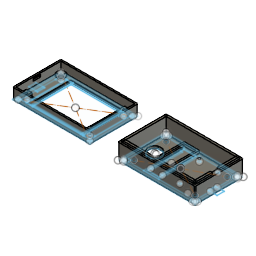
dcdc_cases (Autodesk Fusion 360 design; units mm, degrees)
part number: 2026-03-09-11-10-45-876
Autodesk Fusion 360 part; units mm, degrees
sketch "Sketch1" plane through (0, 0, 0) normal (0, 1, 0) x (1, 0, 0)
  line L0 (0, 0) -> (30.8, 0)
  line L1 (30.8, 0) -> (30.8, 45.2)
  line L2 (30.8, 45.2) -> (0, 45.2)
  line L3 (0, 45.2) -> (0, 0)
  line L4 (0, 0) -> (30.8, 0)
  line L5 (30.8, 0) -> (30.8, 37.2)
  line L6 (30.8, 37.2) -> (0, 37.2)
  line L7 (0, 37.2) -> (0, 0)
  line L8 (0, 45.2) -> (3.78, 45.2)
  line L9 (0, 41.42) -> (0, 45.2)
  circle A0 centre (3.78, 41.42) radius 1.85
  circle A1 centre (27, 41.42) radius 1.85
  line L10 (15.4, 0) -> (0, 0)
  line L11 (0, 0) -> (0, 5.5)
  circle A2 centre (15.4, 5.5) radius 2
  circle A3 centre (15.4, 5.5) radius 3
  line L12 (-1.5, 0) -> (-1.5, 45.2)
  line L13 (-1.5, 45.2) -> (0, 45.2)
  line L14 (0, 45.2) -> (0, 0)
  line L15 (32.3, 0) -> (32.3, 45.2)
  line L16 (32.3, 45.2) -> (30.8, 45.2)
  line L17 (30.8, 45.2) -> (30.8, 0)
  line L18 (32.3, 0) -> (32.3, -1.5)
  line L19 (32.3, -1.5) -> (-1.5, -1.5)
  line L20 (-1.5, -1.5) -> (-1.5, 0)
  circle A4 centre (40.4187, 7.745) radius 3
  circle A5 centre (40.4187, 7.745) radius 2
  line L21 (30.8, 44.0804) -> (30.8, 41.0217)
  line L22 (-1.5, 45.2) -> (32.3, 45.2)
  line L23 (32.3, 45.2) -> (32.3, -1.5)
  line L24 (32.3, -1.5) -> (-1.5, -1.5)
  line L25 (-1.5, -1.5) -> (-1.5, 45.2)
  circle A6 centre (40.4187, 7.745) radius 3
  line L26 (15.4, 0) -> (0, 0)
  line L27 (30.8, 0) -> (30.8, 45.2)
  line L28 (30.8, 44.0804) -> (30.8, 41.0217)
  line L29 (32.3, 0) -> (32.3, 45.2)
  line L30 (30.8, 0) -> (30.8, 37.2)
  line L31 (32.3, 45.2) -> (30.8, 45.2)
  line L32 (30.8, 45.2) -> (0, 45.2)
  line L33 (32.3, 0) -> (32.3, -1.5)
  line L34 (0, 0) -> (30.8, 0)
  line L35 (30.8, 45.2) -> (30.8, 0)
  circle A7 centre (15.4, 5.5) radius 2
  line L36 (30.8, 37.2) -> (0, 37.2)
  line L37 (32.3, 45.2) -> (32.3, -1.5)
  line L38 (0, 0) -> (0, 5.5)
  line L39 (-1.5, 45.2) -> (32.3, 45.2)
  line L40 (0, 37.2) -> (0, 0)
  line L41 (32.3, -1.5) -> (-1.5, -1.5)
  line L42 (0, 0) -> (30.8, 0)
  line L43 (32.3, -1.5) -> (-1.5, -1.5)
  line L44 (-1.5, -1.5) -> (-1.5, 45.2)
  line L45 (-1.5, 0) -> (-1.5, 45.2)
  line L46 (0, 45.2) -> (0, 0)
  circle A8 centre (40.4187, 7.745) radius 2
  line L47 (0, 45.2) -> (0, 0)
  circle A9 centre (27, 41.42) radius 1.85
  circle A10 centre (15.4, 5.5) radius 3
  line L48 (-1.5, -1.5) -> (-1.5, 0)
  circle A11 centre (3.78, 41.42) radius 1.85
  line L49 (0, 41.42) -> (0, 45.2)
  line L50 (0, 45.2) -> (3.78, 45.2)
  line L51 (-1.5, 45.2) -> (0, 45.2)
  dimension "d7" = 3.7
  dimension "d8" = 3.7
  dimension "d10" = 4
  dimension "d11" = 6
  dimension "d12" = 1.5
  dimension "d13" = 1.5
  dimension "d14" = 1.5
  dimension "d50" = 6
  dimension "d51" = 4
  dimension "d79" = 33.8
  dimension "d80" = 46.7
  dimension "d127" = 3.7
  dimension "d128" = 3.7
  dimension "d129" = 4
  dimension "d130" = 6
  dimension "d131" = 1.5
  dimension "d132" = 1.5
  dimension "d133" = 1.5
  dimension "d134" = 6
  dimension "d135" = 4
  dimension "d136" = 33.8
  dimension "d137" = 46.7
  constraint horizontal L0
  constraint vertical L1
  constraint horizontal L2
  constraint vertical L3
  constraint coincident L0.start L3.end
  constraint horizontal L4
  constraint vertical L5
  constraint horizontal L6
  constraint vertical L7
  constraint horizontal L8
  constraint vertical L9
  constraint horizontal L10
  constraint vertical L11
  constraint midpoint L4 L10.start
  constraint concentric A2 A3
  constraint vertical L12
  constraint horizontal L13
  constraint vertical L14
  constraint vertical L15
  constraint horizontal L16
  constraint vertical L17
  constraint vertical L18
  constraint horizontal L19
  constraint vertical L20
  constraint concentric A4 A5
  constraint vertical L21
  constraint coincident L17 L21.end
  constraint horizontal L22
  constraint vertical L23
  constraint horizontal L24
  constraint vertical L25
  constraint horizontal L34
  constraint vertical L27
  constraint horizontal L32
  constraint vertical L46
  constraint horizontal L42
  constraint vertical L30
  constraint horizontal L36
  constraint vertical L40
  constraint horizontal L50
  constraint vertical L49
  constraint horizontal L26
  constraint vertical L38
  constraint midpoint L10.start L42
  constraint concentric A7 A10
  constraint vertical L45
  constraint horizontal L51
  constraint vertical L47
  constraint vertical L29
  constraint horizontal L31
  constraint vertical L35
  constraint vertical L33
  constraint horizontal L43
  constraint vertical L48
  constraint concentric A6 A8
  constraint vertical L28
  constraint coincident L21.end L35
  constraint horizontal L39
  constraint vertical L37
  constraint horizontal L41
  constraint vertical L44
  measures "d7" diameter of A0
  measures "d8" diameter of A1
  measures "d10" diameter of A2
  measures "d11" diameter of A3
  measures "d12" distance of L0.start L12.start
  measures "d13" distance of L0.end L15.start
  measures "d14" distance of L12.start L19.end
  measures "d50" diameter of A4
  measures "d51" diameter of A5
  measures "d79" distance of L18.end L19.end
  measures "d80" distance of L12.end L19.end
  measures "d127" diameter of A11
  measures "d128" diameter of A9
  measures "d129" diameter of A7
  measures "d130" diameter of A10
  measures "d131" distance of L0.start L12.start
  measures "d132" distance of L0.end L15.start
  measures "d133" distance of L19.end L12.start
  measures "d134" diameter of A6
  measures "d135" diameter of A8
  measures "d136" distance of L19.end L18.end
  measures "d137" distance of L19.end L12.end
extrude "Extrude1" add sketch "Sketch1" along normal blind 1.5 contours L0 L1 L3 L4 L5 L6 L7 L10 L11 L14 L17 L26 L27 L30 L34 L35 L36 L38 L40 L42 L46 L47 | L1 L2 L3 L6 L8 L9 L14 L17 L21 L22 L27 L28 L32 L35 L36 L39 L46 L47 L49 L50 | A3 A10 makes body 1
extrude "Extrude2" add sketch "Sketch1" along normal blind 17.7 contours L0 L1 L3 L4 L5 L7 L9 L10 L11 L12 L13 L14 L15 L16 L17 L18 L19 L20 L21 L22 L23 L24 L25 L26 L27 L28 L29 L30 L31 L33 L34 L35 L37 L38 L39 L40 L41 L42 L43 L44 L45 L46 L47 L48 L49 L51 bodies 1
ref_plane "WorkPlane1" through (15.4, 17.7, -21.85) normal (0, 1, 0) x (0, 0, 1)
sketch "Sketch2" plane through (0, 17.7, 0) normal (0, 1, 0) x (1, 0, 0)
  line L0 (-1.5, -1.5) -> (32.3, -1.5)
  line L1 (32.3, -1.5) -> (32.3, 37.2)
  line L2 (32.3, 37.2) -> (-1.5, 37.2)
  line L3 (-1.5, 37.2) -> (-1.5, -1.5)
  circle A0 centre (15.4, 5.5) radius 2
  circle A1 centre (15.4, 5.5) radius 3
  dimension "d20" = 4
  dimension "d21" = 6
  constraint horizontal L0
  constraint vertical L1
  constraint horizontal L2
  constraint vertical L3
  constraint concentric A0 A1
  measures "d20" diameter of A0
  measures "d21" diameter of A1
extrude "Extrude3" add sketch "Sketch2" along normal blind 1.5 contours L0 L1 L2 L3 bodies 1
fillet "Fillet1" radius 1 2 edges at (31.55, 17.7, -37.2) (-0.75, 17.7, -37.2) on bodies 1
fillet "Fillet2" radius 2 2 edges at (-0.75, 17.7, -45.2) (31.55, 17.7, -45.2) on bodies 1
sketch "mini-170" plane through (0, 0, 0) normal (0, 1, 0) x (1, 0, 0)
  line L0 (0, 0) -> (10.9, 0)
  line L1 (10.9, 0) -> (10.9, 20.2)
  line L2 (0, 20.2) -> (0, 0)
  line L3 (-1.5, 20.2) -> (-1.5, 0)
  line L4 (0, 0) -> (0, 20.2)
  line L5 (12.4, 20.2) -> (12.4, 0)
  line L6 (10.9, 0) -> (10.9, 20.2)
  line L7 (12.4, 0) -> (12.4, -1.5)
  line L8 (12.4, -1.5) -> (-1.5, -1.5)
  line L9 (-1.5, -1.5) -> (-1.5, 0)
  line L10 (-1.5, 9.9832) -> (-1.5, 11.0323)
  line L11 (-6.4986, 11.0323) -> (-6.4986, 9.9832)
  line L12 (12.4, 10.1) -> (12.4, 11.4359)
  circle A0 centre (-3.9993, 9.9832) radius 1.5
  circle A1 centre (14.9, 10.1) radius 1.5
  arc A2 (-1.5, 15.1) -> (-1.5, 5.1) centre (-1.5, 10.1) ccw
  arc A3 (12.4, 5.1) -> (12.4, 15.1) centre (12.4, 10.1) ccw
  line L13 (12.4, 20.2) -> (12.4, 23.2)
  line L14 (12.4, 23.2) -> (-1.5, 23.2)
  line L15 (-1.5, 23.2) -> (-1.5, 20.2)
  line L16 (-1.5, 20.2) -> (-1.5, 23.2)
  line L17 (-1.5, 23.2) -> (0, 23.2)
  line L18 (0, 23.2) -> (0, 20.2)
  line L19 (12.4, 20.2) -> (12.4, 23.2)
  line L20 (12.4, 23.2) -> (10.9, 23.2)
  line L21 (10.9, 23.2) -> (10.9, 20.2)
  constraint horizontal L0
  constraint vertical L1
  constraint vertical L2
  constraint coincident L0.start L2.end
  constraint vertical L3
  constraint vertical L4
  constraint vertical L5
  constraint vertical L6
  constraint vertical L7
  constraint horizontal L8
  constraint vertical L9
  constraint midpoint L5 L12.start
  constraint midpoint L3 A2.centre
  constraint vertical L10
  constraint vertical L11
  constraint coincident L3 L10.end
  constraint coincident L11.end A2
  constraint vertical L12
  constraint coincident L5 L12.end
  constraint coincident L3 A2.start
  constraint coincident L3 A2.end
  constraint coincident L5 A3.start
  constraint coincident L5 A3.end
  constraint vertical L13
  constraint horizontal L14
  constraint vertical L15
  constraint vertical L16
  constraint horizontal L17
  constraint vertical L18
  constraint vertical L19
  constraint horizontal L20
  constraint vertical L21
extrude "Extrude5" add sketch "mini-170" along normal blind 1.5 separate body contours L0 L1 L2 L4 L6 L14 L18 L21 makes body 2
extrude "Extrude6" add sketch "mini-170" along normal blind 6.1 contours L0 L1 L2 L3 L4 L5 L6 L7 L8 L9 L10 L12 L13 L14 L15 L16 L17 L18 L19 L20 L21 bodies 2
ref_plane "WorkPlane2" through (5.45, 6.1, -10.85) normal (0, 1, 0) x (0, 0, 1)
sketch "mini-170_top" plane through (0, 6.1, 0) normal (0, 1, 0) x (1, 0, 0)
  line L0 (-1.5, -1.5) -> (12.4, -1.5)
  line L1 (12.4, -1.5) -> (12.4, 23.2)
  line L2 (12.4, 23.2) -> (-1.5, 23.2)
  line L3 (-1.5, 23.2) -> (-1.5, -1.5)
  dimension "d45" = 13.9
  constraint horizontal L0
  constraint vertical L1
  constraint horizontal L2
  constraint vertical L3
  measures "d45" distance of L0.start L0.end
extrude "Extrude7" add sketch "mini-170_top" along normal blind 1.5 bodies 2
extrude "Extrude8" add sketch "mini-170" along normal blind 4 contours L3 L10 A2 | L5 L12 A3 bodies 2
extrude "Extrude9" add sketch "Sketch1" along normal blind 15.3 separate body contours A4 A6 makes body 3
sketch "esp_main_board" plane through (0, 0, 0) normal (0, 1, 0) x (1, 0, 0)
  line L0 (91.015, 60.1) -> (-4.985, 60.1)
  line L1 (0, 32.65) -> (0, 23.8)
  line L2 (2, 32.65) -> (0, 32.65)
  circle A0 centre (87.5225, 3.55) radius 1.25
  line L3 (74.83, 55.2) -> (77.53, 55.2)
  circle A1 centre (4, 9) radius 0.9
  line L4 (74.83, 7.7) -> (14.9, 7.7)
  line L5 (0, 55.2) -> (-2.985, 55.2)
  circle A2 centre (87.5225, 56.65) radius 1.25
  line L6 (-2.985, 58.1) -> (0, 58.1)
  line L7 (86.03, 5) -> (77.53, 5)
  line L8 (14.9, 5) -> (74.83, 5)
  line L9 (89.015, 2.1) -> (89.015, 58.1)
  line L10 (77.53, 5) -> (77.53, 55.2)
  line L11 (77.53, 5) -> (74.83, 5)
  line L12 (2, 23.8) -> (2, 32.65)
  line L13 (0, 55.2) -> (0, 5)
  line L14 (77.53, 5) -> (77.53, 55.2)
  line L15 (14.9, 5) -> (14.9, 55.2)
  line L16 (0, 5) -> (-2.985, 5)
  line L17 (86.03, 5) -> (0, 5)
  line L18 (7.03, 5) -> (77.53, 5)
  line L19 (-2.985, 2.1) -> (89.015, 58.1) construction
  circle A3 centre (82.03, 9) radius 0.9
  line L20 (91.015, 0.1) -> (-4.985, 60.1) construction
  line L21 (89.015, 55.2) -> (89.015, 58.1)
  line L22 (-4.985, 0.1) -> (91.015, 0.1)
  line L23 (7.6, 5) -> (14.9, 5)
  line L24 (91.015, 0.1) -> (91.015, 60.1)
  line L25 (14.9, 52.5) -> (14.9, 55.2)
  line L26 (89.015, 2.1) -> (-2.985, 58.1) construction
  line L27 (-2.985, 2.1) -> (89.015, 2.1)
  line L28 (89.015, 2.1) -> (86.03, 2.1)
  line L29 (86.03, 55.2) -> (89.015, 55.2)
  line L30 (86.03, 58.1) -> (86.03, 55.2)
  line L31 (86.03, 2.1) -> (86.03, 5)
  line L32 (77.53, 55.2) -> (77.53, 5)
  line L33 (74.83, 52.5) -> (14.9, 52.5)
  circle A4 centre (82.03, 51.2) radius 0.9
  line L34 (86.03, 55.2) -> (86.03, 5)
  line L35 (74.83, 55.2) -> (74.83, 52.5)
  line L36 (0, 2.1) -> (0, 5)
  line L37 (89.015, 5) -> (89.015, 2.1)
  line L38 (77.53, 55.2) -> (86.03, 55.2)
  line L39 (89.015, 58.1) -> (86.03, 58.1)
  line L40 (86.03, 55.2) -> (86.03, 5)
  line L41 (74.83, 5) -> (74.83, 7.7)
  line L42 (89.015, 58.1) -> (-2.985, 58.1)
  line L43 (0, 58.1) -> (0, 55.2)
  line L44 (7.6, 5) -> (7.6, 55.2)
  line L45 (86.03, 5) -> (89.015, 5)
  line L46 (14.9, 7.7) -> (14.9, 5)
  circle A5 centre (-1.4925, 56.65) radius 1.25
  line L47 (0, 5) -> (7.6, 5)
  line L48 (-2.985, 55.2) -> (-2.985, 58.1)
  line L49 (-2.985, 5) -> (-2.985, 2.1)
  circle A6 centre (4, 51.2) radius 0.9
  line L50 (74.83, 5) -> (74.83, 55.2)
  circle A7 centre (-1.4925, 3.55) radius 1.25
  line L51 (7.03, 55.2) -> (7.03, 5)
  line L52 (-2.985, 2.1) -> (0, 2.1)
  line L53 (14.9, 55.2) -> (74.83, 55.2)
  line L54 (-4.985, 60.1) -> (-4.985, 0.1)
  line L55 (7.6, 55.2) -> (0, 55.2)
  line L56 (-2.985, 58.1) -> (-2.985, 2.1)
  line L57 (7.6, 55.2) -> (7.6, 5)
  line L58 (0, 23.8) -> (2, 23.8)
  line L59 (77.53, 55.2) -> (7.03, 55.2)
  line L60 (-4.985, 0.1) -> (91.015, 60.1) construction
  line L61 (14.9, 55.2) -> (7.6, 55.2)
  line L62 (0, 5) -> (7.03, 5)
  line L63 (7.03, 5) -> (7.03, 12)
  line L64 (7.03, 12) -> (0, 12)
  line L65 (0, 12) -> (0, 5)
  line L66 (0, 55.2) -> (7.03, 55.2)
  line L67 (7.03, 55.2) -> (7.03, 48.2)
  line L68 (7.03, 48.2) -> (0, 48.2)
  line L69 (0, 48.2) -> (0, 55.2)
  line L70 (86.03, 55.2) -> (79.03, 55.2)
  line L71 (79.03, 55.2) -> (79.03, 48.2)
  line L72 (79.03, 48.2) -> (86.03, 48.2)
  line L73 (86.03, 48.2) -> (86.03, 55.2)
  line L74 (86.03, 5) -> (79.03, 5)
  line L75 (79.03, 5) -> (79.03, 12)
  line L76 (79.03, 12) -> (86.03, 12)
  line L77 (86.03, 12) -> (86.03, 5)
  line L78 (2, 23.8) -> (-8.6658, 23.8)
  line L79 (-8.6658, 23.8) -> (-8.6658, 32.65)
  line L80 (-8.6658, 32.65) -> (2, 32.65)
  line L81 (2, 32.65) -> (2, 23.8)
  line L82 (14.9, 55.2) -> (12.2, 55.2)
  line L83 (12.2, 55.2) -> (12.2, 5)
  line L84 (12.2, 5) -> (14.9, 5)
  line L85 (14.9, 5) -> (14.9, 55.2)
  line L86 (14.9, 53.85) -> (76.18, 53.85)
  line L87 (14.9, 53.85) -> (13.55, 53.85)
  line L88 (14.9, 6.35) -> (76.18, 6.35)
  line L89 (14.9, 6.35) -> (13.55, 6.35)
  line L90 (13.55, 6.35) -> (76.18, 6.35)
  line L91 (76.18, 6.35) -> (76.18, 53.85)
  line L92 (13.55, 53.85) -> (13.55, 6.35)
  line L93 (126.015, 0.1) -> (126.015, 60.1)
  line L94 (222.015, 60.1) -> (222.015, 0.1)
  line L95 (138.8674, 22.8706) -> (144.6215, 22.8706)
  line L96 (131, 2.1) -> (131, 5)
  line L97 (131, 58.1) -> (131, 55.2)
  line L98 (131, 5) -> (128.015, 5)
  line L99 (131, 55.2) -> (128.015, 55.2)
  arc A8 (144.6215, 22.8706) -> (144.6215, 37.3706) centre (141.7444, 30.1206) ccw
  line L100 (126.015, 60.1) -> (222.015, 60.1)
  line L101 (222.015, 0.1) -> (126.015, 0.1)
  arc A9 (138.8674, 37.3706) -> (138.8674, 22.8706) centre (141.7444, 30.1206) ccw
  line L102 (144.6215, 37.3706) -> (138.8674, 37.3706)
  circle A10 centre (201.25, 49.42) radius 1.45
  line L103 (225.6958, 23.8) -> (225.6958, 32.65)
  line L104 (215.03, 23.8) -> (225.6958, 23.8)
  line L105 (225.6958, 32.65) -> (215.03, 32.65)
  circle A11 centre (178.03, 49.42) radius 1.45
  circle A12 centre (189.63, 13.5) radius 1.45
  line L106 (217.03, 5) -> (220.015, 5)
  line L107 (215.03, 32.65) -> (217.03, 32.65)
  line L108 (217.03, 2.1) -> (217.03, 5)
  line L109 (217.03, 23.8) -> (215.03, 23.8)
  line L110 (215.03, 23.8) -> (215.03, 32.65)
  line L111 (215.03, 32.65) -> (215.03, 23.8)
  line L112 (217.03, 58.1) -> (217.03, 55.2)
  line L113 (217.03, 55.2) -> (220.015, 55.2)
  line L114 (170, 53) -> (155.3, 53)
  line L115 (155.3, 53) -> (155.3, 7.5)
  line L116 (155.3, 7.5) -> (170, 7.5)
  line L117 (170, 7.5) -> (170, 53)
  line L118 (130.815, 55.3) -> (217.215, 55.3)
  line L119 (217.215, 55.3) -> (217.215, 4.9)
  line L120 (217.215, 4.9) -> (130.815, 4.9)
  line L121 (130.815, 4.9) -> (130.815, 55.3)
  line L122 (128.09, 58.025) -> (219.94, 58.025)
  line L123 (219.94, 58.025) -> (219.94, 2.175)
  line L124 (219.94, 2.175) -> (128.09, 2.175)
  line L125 (128.09, 2.175) -> (128.09, 58.025)
  line L126 (128.09, 58.025) -> (134.09, 58.025)
  line L127 (134.09, 58.025) -> (134.09, 52.025)
  line L128 (134.09, 52.025) -> (128.09, 52.025)
  line L129 (128.09, 52.025) -> (128.09, 58.025)
  line L130 (128.09, 2.175) -> (134.09, 2.175)
  line L131 (134.09, 2.175) -> (134.09, 8.175)
  line L132 (134.09, 8.175) -> (128.09, 8.175)
  line L133 (128.09, 8.175) -> (128.09, 2.175)
  line L134 (219.94, 58.025) -> (213.94, 58.025)
  line L135 (213.94, 58.025) -> (213.94, 52.025)
  line L136 (213.94, 52.025) -> (219.94, 52.025)
  line L137 (219.94, 52.025) -> (219.94, 58.025)
  line L138 (219.94, 2.175) -> (213.94, 2.175)
  line L139 (213.94, 2.175) -> (213.94, 8.175)
  line L140 (213.94, 8.175) -> (219.94, 8.175)
  line L141 (219.94, 8.175) -> (219.94, 2.175)
  line L142 (172.15, 4.9) -> (153.15, 4.9)
  line L143 (153.15, 4.9) -> (153.15, 55.3)
  line L144 (172.15, 55.3) -> (172.15, 4.9)
  line L145 (155.3, 53) -> (170, 53)
  line L146 (170, 53) -> (170, 49)
  line L147 (155.3, 49) -> (155.3, 53)
  line L148 (155.3, 7.5) -> (170, 7.5)
  line L149 (170, 7.5) -> (170, 11.5)
  line L150 (155.3, 11.5) -> (155.3, 7.5)
  line L151 (155.3, 49) -> (157.3, 49)
  line L152 (157.3, 49) -> (157.3, 11.5)
  line L153 (157.3, 11.5) -> (155.3, 11.5)
  line L154 (155.3, 11.5) -> (155.3, 49)
  line L155 (170, 49) -> (168, 49)
  line L156 (168, 49) -> (168, 11.5)
  line L157 (168, 11.5) -> (170, 11.5)
  line L158 (170, 11.5) -> (170, 49)
  circle A13 centre (129.5075, 56.65) radius 1.4
  circle A14 centre (218.5225, 56.65) radius 1.4
  circle A15 centre (129.5075, 3.55) radius 1.4
  circle A16 centre (218.5225, 3.55) radius 1.45
  line L159 (212.015, 10.1) -> (136.015, 50.1) construction
  line L160 (136.015, 10.1) -> (212.015, 50.1) construction
  circle A17 centre (136.015, 50.1) radius 2
  circle A18 centre (136.015, 10.1) radius 2
  circle A19 centre (212.015, 10.1) radius 2
  circle A20 centre (212.015, 50.1) radius 2
  point P0 (43.015, 30.1)
  point P1 (43.015, 30.1)
  point P2 (0, 55.2)
  point P3 (217.03, 55.2)
  point P4 (143.7444, 30.1206)
  point P5 (205.03, 8)
  point P6 (174.015, 30.1)
  point P7 (174.015, 30.1)
  point P8 (174.015, 30.1)
  point P9 (174.015, 30.1)
  point P10 (162.65, 30.25)
  point P11 (174.015, 30.1)
  dimension "d95" = 7
  dimension "d96" = 7
  dimension "d98" = 7
  dimension "d99" = 7
  dimension "d100" = 7
  dimension "d103" = 1.8
  dimension "d104" = 1.8
  dimension "d105" = 1.8
  dimension "d106" = 1.8
  dimension "d202" = 2.8
  dimension "d203" = 2.8
  dimension "d205" = 2.8
  dimension "d206" = 2.9
  dimension "d225" = 2.9
  dimension "d226" = 2.9
  dimension "d227" = 2.9
  dimension "d236" = 76
  dimension "d237" = 40
  dimension "d238" = 4
  dimension "d239" = 4
  dimension "d240" = 4
  dimension "d241" = 4
  constraint horizontal L62
  constraint vertical L63
  constraint horizontal L64
  constraint vertical L65
  constraint horizontal L66
  constraint vertical L67
  constraint horizontal L68
  constraint vertical L69
  constraint coincident P2 L5.start
  constraint horizontal L70
  constraint vertical L71
  constraint horizontal L72
  constraint vertical L73
  constraint horizontal L74
  constraint vertical L75
  constraint horizontal L76
  constraint vertical L77
  constraint horizontal L78
  constraint vertical L79
  constraint horizontal L80
  constraint vertical L81
  constraint horizontal L82
  constraint vertical L83
  constraint horizontal L84
  constraint vertical L85
  constraint midpoint L25 L86.start
  constraint perpendicular L10 L86
  constraint perpendicular L83 L87
  constraint midpoint L46 L88.start
  constraint perpendicular L32 L88
  constraint perpendicular L85 L89
  constraint perpendicular L10 L90
  constraint perpendicular L3 L91
  constraint perpendicular L17 L92
  constraint symmetric L101.end L93 L93.start
  constraint horizontal L114
  constraint vertical L115
  constraint horizontal L116
  constraint horizontal L118
  constraint perpendicular L118 L119
  constraint parallel L118 L120
  constraint parallel L119 L121
  constraint coincident P11 P9
  constraint horizontal L122
  constraint perpendicular L122 L123
  constraint parallel L122 L124
  constraint parallel L123 L125
  constraint horizontal L126
  constraint vertical L127
  constraint horizontal L128
  constraint vertical L129
  constraint horizontal L130
  constraint vertical L131
  constraint horizontal L132
  constraint vertical L133
  constraint horizontal L134
  constraint vertical L135
  constraint horizontal L136
  constraint vertical L137
  constraint horizontal L138
  constraint vertical L139
  constraint horizontal L140
  constraint vertical L141
  constraint horizontal L142
  constraint perpendicular L142 L143
  constraint parallel L143 L144
  constraint coincident L118 L143.end
  constraint coincident L118 L144.start
  constraint horizontal L145
  constraint vertical L146
  constraint vertical L147
  constraint coincident L117 L146.end
  constraint horizontal L148
  constraint vertical L149
  constraint vertical L150
  constraint horizontal L151
  constraint vertical L152
  constraint horizontal L153
  constraint vertical L154
  constraint horizontal L155
  constraint vertical L156
  constraint horizontal L157
  constraint vertical L158
  constraint coincident L159 P11
  constraint coincident L160 P11
  constraint coincident L159.end A17.centre
  constraint coincident L160.start A18.centre
  constraint coincident L159.start A19.centre
  constraint coincident L160.end A20.centre
  measures "d95" distance of L13.end L64.end
  measures "d96" distance of P2 L68.end
  measures "d98" distance of L29.start L72.end
  measures "d99" distance of L7.start L74.end
  measures "d100" distance of L7.start L76.end
  measures "d103" diameter of A6
  measures "d104" diameter of A4
  measures "d105" diameter of A1
  measures "d106" diameter of A3
  measures "d202" diameter of A13
  measures "d203" diameter of A14
  measures "d205" diameter of A15
  measures "d206" diameter of A16
  measures "d225" diameter of A11
  measures "d226" diameter of A10
  measures "d227" diameter of A12
  measures "d236" distance of L159.end L160.end
  measures "d237" distance of L160.start L159.end
  measures "d238" diameter of A17
  measures "d239" diameter of A18
  measures "d240" diameter of A19
  measures "d241" diameter of A20
extrude "Extrude10" add sketch "esp_main_board" along normal blind 3 separate body contours L0 L6 L9 L21 L22 L24 L27 L28 L37 L39 L42 L48 L49 L52 L54 L56 L78 L80 | L54 L56 L78 L80 | L1 L13 L56 L78 L80 | L5 L13 L56 L69 L80 | L13 L16 L56 L65 L78 | L5 L6 L42 L43 L48 L56 | L1 L2 L12 L13 L58 L78 L80 L81 | L2 L12 L13 L51 L58 L64 L68 L78 L80 L81 | L16 L27 L36 L49 L52 L56 | L13 L51 L55 L66 L67 L68 L69 | L3 L30 L38 L42 L43 L53 L55 L59 L61 L66 L70 L82 | L13 L17 L47 L51 L62 L63 L64 L65 | L7 L8 L11 L17 L18 L23 L27 L31 L36 L47 L62 L74 L84 | L17 L18 L44 L47 L51 L55 L57 L59 L63 L67 | L9 L21 L29 L30 L39 L42 | L17 L18 L23 L44 L57 L59 L61 L83 | L9 L27 L28 L31 L37 L45 | L9 L29 L34 L40 L45 L73 L77 | L34 L38 L40 L70 L71 L72 L73 | L15 L17 L18 L23 L25 L46 L59 L61 L82 L83 L84 L85 L87 L89 L90 L92 | L7 L17 L34 L40 L74 L75 L76 L77 | L7 L10 L14 L17 L32 L34 L38 L40 L71 L72 L75 L76 | L15 L25 L35 L50 L53 L59 L85 L86 | L8 L15 L17 L18 L41 L46 L50 L85 L88 L90 | L3 L10 L11 L14 L17 L18 L32 L35 L41 L50 L59 L86 L88 L90 L91 | L15 L25 L33 L35 L50 L85 L86 | L15 L25 L46 L85 L87 L89 L90 L92 | L4 L15 L41 L46 L50 L85 L88 L90 | L35 L41 L50 L86 L88 L90 L91 | A1 | A3 | A4 | A6 makes body 4
extrude "Extrude11" add sketch "esp_main_board" along normal blind 7.4 contours L13 L51 L55 L66 L67 L68 L69 | L13 L17 L47 L51 L62 L63 L64 L65 | L34 L38 L40 L70 L71 L72 L73 | L7 L17 L34 L40 L74 L75 L76 L77 bodies 4
extrude "Extrude12" add sketch "esp_main_board" along normal blind 13.4 contours L0 L6 L9 L21 L22 L24 L27 L28 L37 L39 L42 L48 L49 L52 L54 L56 L78 L80 | L54 L56 L78 L80 bodies 4
ref_plane "WorkPlane3" through (-4.985, 6.7, -30.1) normal (-1, 0, 0) x (0, 0, 1)
sketch "esp_usb" plane through (-4.985, 0, 0) normal (-1, 0, 0) x (0, 0, 1)
  line L0 (-32.65, 0) -> (-23.8, 0)
  line L1 (-32.65, 0) -> (-23.8, 0)
  line L2 (-23.8, 0) -> (-23.8, 8.95)
  line L3 (-23.8, 8.95) -> (-32.65, 8.95)
  line L4 (-32.65, 8.95) -> (-32.65, 0)
  line L5 (-32.65, 8.95) -> (-23.8, 8.95)
  line L6 (-23.8, 8.95) -> (-23.8, 12.15)
  line L7 (-23.8, 12.15) -> (-32.65, 12.15)
  line L8 (-32.65, 12.15) -> (-32.65, 8.95)
  dimension "d113" = 8.95
  dimension "d114" = 3.2
  constraint horizontal L0
  constraint horizontal L1
  constraint vertical L2
  constraint horizontal L3
  constraint vertical L4
  constraint horizontal L5
  constraint vertical L6
  constraint horizontal L7
  constraint vertical L8
  measures "d113" distance of L0.start L3.end
  measures "d114" distance of L3.end L7.end
extrude "Extrude14" cut sketch "esp_usb" against normal up to surface (2 mm away) contours L3 L5 L6 L7 L8 bodies 4
ref_plane "WorkPlane4" through (43.015, 3, -30.1) normal (0, 1, 0) x (1, 0, 0)
sketch "esp32_rubber" plane through (0, 3, 0) normal (0, 1, 0) x (1, 0, 0)
  line L0 (13.55, 53.85) -> (13.55, 6.35)
  line L1 (14.9, 53.85) -> (76.18, 53.85)
  line L2 (14.9, 53.85) -> (13.55, 53.85)
  line L3 (76.18, 6.35) -> (76.18, 53.85)
  line L4 (13.55, 6.35) -> (76.18, 6.35)
pipe "Pipe1" cut diameter 1 path "esp32_rubber" along L1 L3 L4 L0 L2 bodies 4
fillet "Fillet3" radius 2 4 edges at (44.865, 0, -7.7) (74.83, 0, -30.1) (44.865, 0, -52.5) (14.9, 0, -30.1) on bodies 4
fillet "Fillet4" radius 1 4 edges at (-4.985, 6.7, -0.1) (-4.985, 6.7, -60.1) (91.015, 6.7, -0.1) (91.015, 6.7, -60.1) on bodies 4
extrude "Extrude16" add sketch "esp_main_board" along normal blind 3 separate body contours L93 L94 L100 L101 L104 L105 L122 L123 L124 L125 L126 L129 L130 L133 L134 L137 L138 L141 A13 A14 A15 A16 | L94 L104 L105 L123 | L104 L119 L123 L140 | L104 L105 L119 L123 | L105 L119 L123 L136 | L104 L105 L107 L109 L110 L111 L118 L119 L120 L135 L136 L139 L140 L144 | L104 L105 L107 L109 L110 L111 L119 | L106 L119 L123 L140 L141 | L113 L119 L123 L136 L137 | L106 L108 L119 L120 L139 L140 | L106 L123 L141 A16 | L112 L113 L118 L119 L135 L136 | L112 L113 L118 L119 L122 L123 L134 L137 A14 | L106 L108 L119 L120 | L106 L108 L119 L120 L124 L138 A16 | L123 L124 L138 L141 A16 | L123 L141 A16 | L112 L113 L118 L119 | L120 L124 L131 L139 L142 | L108 L120 L124 L138 L139 | L124 L138 A16 | L123 L124 L138 L141 A16 | L112 L118 L122 L134 L135 | L118 L122 L127 L135 | L122 L134 A14 | L122 L134 A14 | L118 L120 L142 L143 L144 | L118 L120 L121 L127 L128 L131 L132 L143 | L96 L120 L124 L130 L131 | L97 L118 L122 L126 L127 | L96 L98 L120 L121 L131 L132 | L96 L98 L120 L121 L124 L125 L130 L133 A15 | L97 L99 L118 L121 L127 L128 | L97 L99 L118 L121 L122 L125 L126 L129 A13 | L96 L98 L120 L121 | L124 L130 A15 | L124 L130 A15 | L97 L99 L118 L121 | L122 L126 A13 | L122 L126 A13 | L121 L125 L128 L132 | L98 L121 L125 L132 L133 | L99 L121 L125 L128 L129 | L95 A8 A9 L102 | A10 | A11 | A12 | L114 L115 L116 L117 L145 L146 L147 L148 L149 L150 L151 L152 L153 L155 L156 L157 | L117 L155 L156 L157 L158 | L115 L151 L152 L153 L154 | A17 | A18 | A19 | A20 makes body 5
extrude "Extrude18" add sketch "esp_main_board" along normal blind 22 separate body contours L104 L119 L123 L140 | L104 L105 L119 L123 | L105 L119 L123 L136 | L106 L119 L123 L140 L141 | L113 L119 L123 L136 L137 | L106 L123 L141 A16 | L112 L113 L118 L119 L122 L123 L134 L137 A14 | L106 L108 L119 L120 L124 L138 A16 | L123 L124 L138 L141 A16 | L120 L124 L131 L139 L142 | L108 L120 L124 L138 L139 | L123 L124 L138 L141 A16 | L112 L118 L122 L134 L135 | L118 L122 L127 L135 | L122 L134 A14 | L96 L120 L124 L130 L131 | L97 L118 L122 L126 L127 | L96 L98 L120 L121 L124 L125 L130 L133 A15 | L97 L99 L118 L121 L122 L125 L126 L129 A13 | L124 L130 A15 | L122 L126 A13 | L121 L125 L128 L132 | L98 L121 L125 L132 L133 | L99 L121 L125 L128 L129 picked at (219.2137, 57.0077) picked at (128.9376, 3.9758) picked at (130.3837, 56.9215) makes body 6
extrude "Extrude19" add sketch "esp_main_board" along normal blind 19.75 contours L93 L94 L100 L101 L104 L105 L122 L123 L124 L125 L126 L129 L130 L133 L134 L137 L138 L141 A13 A14 A15 A16 | L94 L104 L105 L123 bodies 5 6
extrude "Extrude20" cut sketch "esp_main_board" along normal blind 22 contours L104 L105 L119 L123 bodies 5
extrude "Extrude21" add sketch "esp_main_board" along normal up to surface (3 mm away) contours L104 L105 L119 L123 bodies 5
extrude "Extrude22" cut sketch "esp_main_board" along normal up to surface (22 mm away) contours L123 L124 L138 L141 A16 | L122 L134 A14 | L124 L130 A15 | L122 L126 A13 picked at (219.0634, 3.1321) picked at (219.2137, 57.0077) picked at (128.9376, 3.9758) picked at (130.3837, 56.9215) bodies 5
extrude "Extrude23" add sketch "esp_main_board" along normal blind 14 contours L123 L124 L138 L141 A16 | L122 L134 A14 | L124 L130 A15 | L122 L126 A13 picked at (219.0634, 3.1321) picked at (219.2137, 57.0077) picked at (128.9376, 3.9758) picked at (130.3837, 56.9215) bodies 5
extrude "Extrude24" add sketch "esp_main_board" along normal blind 6 contours L118 L120 L142 L143 L144 bodies 5
extrude "Extrude25" add sketch "esp_main_board" along normal blind 4 contours L117 L155 L156 L157 L158 | L115 L151 L152 L153 L154 bodies 5
extrude "Extrude26" cut sketch "esp_main_board" along normal up to surface (3 mm away) contours A10 | A11 | A12 bodies 5
extrude "Extrude27" cut sketch "esp_main_board" along normal up to surface (3 mm away) contours L95 A8 A9 L102 bodies 5
extrude "Extrude28" cut sketch "esp_main_board" along normal up to surface (3 mm away) contours A17 | A18 | A19 | A20 bodies 5
fillet "Fillet5" radius 1 4 edges at (126.015, 9.875, -0.1) (126.015, 9.875, -60.1) (222.015, 9.875, -0.1) (222.015, 9.875, -60.1) on bodies 5
ref_plane "WorkPlane5" through (222.015, 9.875, -30.1) normal (1, 0, 0) x (0, 0, -1)
sketch "esp_usb_bot" plane through (222.015, 0, 0) normal (1, 0, 0) x (0, 0, -1)
extrude "Extrude29" add sketch "esp_main_board" along normal blind 19.75 contours L104 L105 L119 L123 bodies 5
hidden bodies 1 2 3
named bodies: "hw-pin", "esp_main_top", "esp_main_bot"
